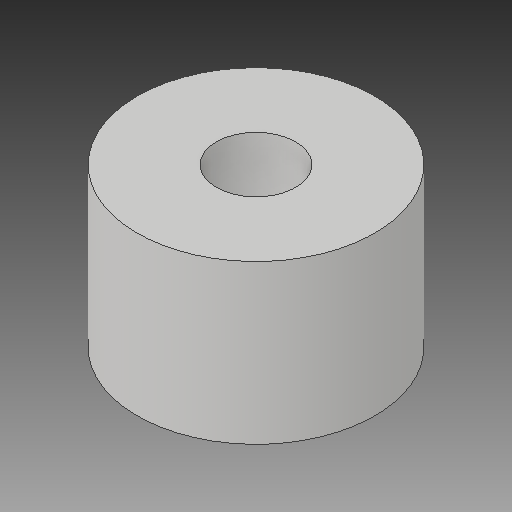
# Autodesk Inventor part: powerDistSpacer
Saved by Autodesk Inventor 2018 (Build 220112000, 112)
## iProperties
Created: 2018-08-04
Part Number: powerDistSpacer
Material: Generic
Document SubType Name: Modeling
Designer: Cole Tucker
Density: 1 g/cm^3
Appearance: Default
Mass: 0.402199 g
Surface Area: 3.80031 cm^2
Volume: 0.402199 cm^3
Author: Cole Tucker
Autodesk Inventor part; units mm, degrees
ref_plane "YZ Plane" through (0, 0, 0) normal (1, 0, 0) x (0, 1, 0)
ref_plane "XZ Plane" through (0, 0, 0) normal (0, 1, 0) x (-1, 0, 0)
ref_plane "XY Plane" through (0, 0, 0) normal (0, 0, 1) x (1, 0, 0)
sketch "Sketch1" plane through (0, 0, 0) normal (0, 1, 0) x (-1, 0, 0)
  circle A0 centre (0, 0) radius 1.5875
  circle A1 centre (0, 0) radius 4.7625
  dimension "d0" = 3.175
  dimension "d1" = 9.525
  constraints: 2 centre point, 2 coincident
  measures "d0" diameter of A0
  measures "d1" diameter of A1
extrude "Extrusion1" add sketch "Sketch1" along normal blind 6.35
body "Solid1"
